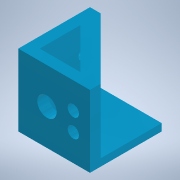
# Autodesk Inventor part: panel connector
Saved by Autodesk Inventor 2020 (Build 240168000, 168)
## iProperties
Created: 2021-02-27
Part Number: panel connector
Material: PC/ABS Plastic
Document SubType Name: Modeling
Designer: Bernard Li
Density: 0.357273 g/cm^3
Appearance: Sky Blue Dark
Author: Bernard Li
Autodesk Inventor part; units mm, degrees
ref_plane "YZ Plane" through (0, 0, 0) normal (1, 0, 0) x (0, 1, 0)
ref_plane "XZ Plane" through (0, 0, 0) normal (0, 1, 0) x (-1, 0, 0)
ref_plane "XY Plane" through (0, 0, 0) normal (0, 0, 1) x (1, 0, 0)
sketch "Sketch1" plane through (0, 0, 0) normal (0, 1, 0) x (-1, 0, 0)
  line L0 (0, 0) -> (-25.4, 0)
  line L1 (-25.4, 0) -> (-25.4, -3.81)
  line L2 (-25.4, -3.81) -> (0, -3.81)
  line L3 (0, -3.81) -> (0, 0)
  line L4 (0, 0) -> (-3.81, 0)
  line L5 (-3.81, 0) -> (-3.81, -25.4)
  line L6 (-3.81, -25.4) -> (0, -25.4)
  line L7 (0, -25.4) -> (0, 0)
  point P0 (-3.81, -3.81)
  dimension "d0" = 25.4
  dimension "d1" = 3.81
  dimension "d2" = 3.81
  dimension "d3" = 25.4
  constraints: 16 end point, 4 parallel, 2 horizontal, 2 perpendicular
  measures "d0" distance of L2.end L1.end
  measures "d1" distance of L1.end L0.end
  measures "d2" distance of L6.end L5.end
  measures "d3" distance of L5.end L4.end
extrude "Extrusion1" add sketch "Sketch1" along normal blind 12.7
sketch "Sketch2" plane through (0, 12.7, 0) normal (0, 1, 0) x (1, 0, 0)
  line L0 (3.81, 3.81) -> (3.81, 25.4) projected
  line L1 (25.4, 3.81) -> (3.81, 3.81) projected
  line L2 (3.81, 25.4) -> (25.4, 3.81)
  line L3 (0, 0) -> (25.4, 0) projected
  line L4 (25.4, 3.81) -> (25.4, 0)
  line L5 (0, 25.4) -> (0, 0) projected
  line L6 (25.4, 0) -> (0, 0)
  line L7 (0, 0) -> (0, 25.4)
  line L8 (0, 25.4) -> (3.81, 25.4)
  constraints: 10 end point, 3 perpendicular, 1 collinear
extrude "Extrusion2" add sketch "Sketch2" along normal blind 6.35
sketch "Sketch3" plane through (0, 0, 0) normal (0, -1, 0) x (1, 0, 0)
  line L0 (3.81, -25.4) -> (0, -25.4) projected
  line L1 (0, -25.4) -> (3.81, -25.4)
  line L2 (25.4, -3.81) -> (3.81, -25.4) projected
  line L3 (3.81, -25.4) -> (25.4, -3.81)
  line L4 (25.4, 0) -> (25.4, -3.81) projected
  line L5 (25.4, -3.81) -> (25.4, 0)
  line L6 (0, 0) -> (25.4, 0) projected
  line L7 (25.4, 0) -> (0, 0)
  line L8 (0, 0) -> (0, -25.4)
  constraints: 10 end point, 2 collinear, 2 perpendicular, 1 horizontal
extrude "Extrusion3" add sketch "Sketch3" along normal blind 6.35
sketch "Sketch4" plane through (0, 12.7, 0) normal (0, -1, 0) x (1, 0, 0)
  line L0 (3.81, -25.4) -> (25.4, -3.81) projected
  line L1 (15.875, -13.335) -> (12.2829, -9.7429)
  line L2 (12.2829, -9.7429) -> (3.81, -18.2158)
  line L3 (3.81, -3.81) -> (3.81, -25.4) projected
  line L4 (25.4, -3.81) -> (3.81, -3.81) projected
  line L5 (3.81, -18.2158) -> (3.81, -3.81)
  line L6 (3.81, -3.81) -> (18.2158, -3.81)
  line L7 (12.2829, -9.7429) -> (18.2158, -3.81)
  dimension "d10" = 5.08
  constraints: 10 end point, 4 point on line, 2 perpendicular, 1 vertical
  measures "d10" distance of L1.start L1.end
extrude "Extrusion4" cut sketch "Sketch4" against normal mid plane 50.8 contours L3 L4 L7 L2
sketch "Sketch5" plane through (3.81, -6.35, -3.81) normal (1, 0, 0) x (0, 0, -1)
  line L0 (0, 6.35) -> (0, 19.05) projected
  line L1 (0, 12.7) -> (21.59, 12.7)
  line L2 (21.59, 6.35) -> (21.59, 19.05) projected
  circle A0 centre (6.35, 12.7) radius 3.429
  circle A1 centre (15.6845, 16.129) radius 2
  circle A2 centre (15.6845, 9.525) radius 2
  line L3 (9.779, 12.7) -> (21.59, 12.7)
  line L4 (15.6845, 12.7) -> (15.6845, 6.35)
  line L5 (14.4058, 6.35) -> (21.59, 6.35) projected
  line L6 (15.6845, 12.7) -> (15.6845, 19.05)
  line L7 (14.4058, 19.05) -> (21.59, 19.05) projected
  circle A3 centre (6.35, 12.9362) radius 6.35
  dimension "d13" = 6.858
  dimension "d16" = 4
  dimension "d17" = 4
  dimension "d18" = 12.7
  constraints: 8 end point, 5 point on line, 4 midpoint, 3 centre point, 2 perpendicular, 1 coincident, 1 horizontal alignment, 1 tangent, 1 vertical, 2 other
  measures "d16" diameter of A1
  measures "d17" diameter of A2
  measures "d18" diameter of A3
extrude "Extrusion5" cut sketch "Sketch5" against normal blind 12.7 contours A0 L1 | L1 A0 | L4 A2 | A2 L4 | L6 A1 | A1 L6
sketch "Sketch6" plane through (3.81, -6.35, -3.81) normal (0, 0, -1) x (-1, 0, 0)
  line L0 (0, 6.35) -> (0, 19.05)
  line L1 (0, 12.7) -> (21.59, 12.7)
  line L2 (21.59, 6.35) -> (21.59, 19.05)
  circle A0 centre (6.35, 12.7) radius 3.429
  circle A1 centre (15.6845, 16.129) radius 2
  circle A2 centre (15.6845, 9.525) radius 2
  line L3 (9.779, 12.7) -> (21.59, 12.7)
  line L4 (15.6845, 12.7) -> (15.6845, 6.35)
  line L5 (14.4058, 6.35) -> (21.59, 6.35)
  line L6 (15.6845, 12.7) -> (15.6845, 19.05)
  line L7 (14.4058, 19.05) -> (21.59, 19.05)
  circle A3 centre (6.35, 12.9362) radius 6.35
  line L8 (-15.6845, 12.7) -> (-15.6845, 6.35)
  circle A4 centre (-15.6845, 9.525) radius 2
  line L9 (-15.6845, 12.7) -> (-15.6845, 19.05)
  line L10 (-9.779, 12.7) -> (-21.59, 12.7)
  circle A5 centre (-15.6845, 16.129) radius 2
  line L11 (-14.4058, 6.35) -> (-21.59, 6.35)
  line L12 (-21.59, 6.35) -> (-21.59, 19.05)
  line L13 (-14.4058, 19.05) -> (-21.59, 19.05)
  line L14 (0, 12.7) -> (-21.59, 12.7)
  circle A6 centre (-6.35, 12.7) radius 3.429
  circle A7 centre (-6.35, 12.9362) radius 6.35
  dimension "d19" = 6.858
  dimension "d20" = 4
  dimension "d21" = 4
  dimension "d22" = 12.7
  constraints: 30 end point, 14 symmetric about line, 10 point on line, 6 centre point, 4 midpoint, 2 coincident, 2 horizontal alignment, 2 perpendicular, 2 vertical, 1 tangent, 7 other
  measures "d20" diameter of A1
  measures "d21" diameter of A2
  measures "d22" diameter of A3
extrude "Extrusion6" cut sketch "Sketch6" against normal blind 12.7 contours A6 L14 | L14 A6 | A4 L8 | L8 A4 | A5 L9 | L9 A5
sketch "Sketch7" plane through (0, -6.35, 0) normal (0, -1, 0) x (1, 0, 0)
  line L0 (25.4, 0) -> (0, 0) projected
  line L1 (0, 0) -> (25.4, 0)
  line L2 (25.4, 0) -> (25.4, -25.4)
  line L3 (25.4, -25.4) -> (0, -25.4)
  line L4 (0, -25.4) -> (0, 0)
  dimension "d25" = 25.4
  dimension "d26" = 25.4
  constraints: 8 end point, 2 parallel, 1 horizontal, 1 perpendicular
  measures "d25" distance of L2.end L3.end
  measures "d26" distance of L1.end L2.end
extrude "Extrusion7" add sketch "Sketch7" against normal blind 2.54
sketch "Sketch8" plane through (0, -3.81, 0) normal (0, 1, 0) x (1, 0, 0)
  circle A0 centre (10.16, 10.16) radius 6.35
  circle A1 centre (10.16, 10.16) radius 3.175
  line L0 (18.2158, 3.81) -> (3.81, 3.81) projected
  line L1 (3.81, 3.81) -> (3.81, 18.2158) projected
  dimension "d29" = 12.7
  dimension "d30" = 6.35
  constraints: 2 centre point, 2 tangent, 1 coincident
  measures "d29" diameter of A0
  measures "d30" diameter of A1
extrude "Extrusion8" cut sketch "Sketch8" against normal mid plane 10.16 contours A1
extrude "Extrusion9" cut sketch "Sketch8" along normal blind 10.16 contours A0
equation "\"d2\" = d1"
body "Solid1"
